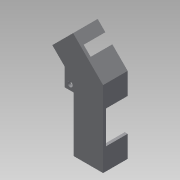
# Autodesk Inventor part: covfronti2c1
Saved by Autodesk Inventor 2015 SP1 (Build 190203100, 203)
## iProperties
Created: 2015-04-15
Part Number: covfronti2c1
Material: Generic
Document SubType Name: Modeling
Designer: Rafi Kurnia Putra
Density: 1 g/cm^3
Appearance: Default
Author: Rafi Kurnia Putra
Autodesk Inventor part; units mm, degrees
ref_plane "YZ Plane" through (0, 0, 0) normal (1, 0, 0) x (0, 1, 0)
ref_plane "XZ Plane" through (0, 0, 0) normal (0, 1, 0) x (-1, 0, 0)
ref_plane "XY Plane" through (0, 0, 0) normal (0, 0, 1) x (1, 0, 0)
sketch "Sketch1" plane through (0, 0, 0) normal (0, 1, 0) x (-1, 0, 0)
  line L0 (-39.6659, 82.3437) -> (-60.406, 61.6036)
  line L1 (-60.406, 61.6036) -> (-60.406, 8.9397)
  circle A0 centre (-37.593, 50.6893) radius 1.75
  circle A1 centre (-37.593, 50.6893) radius 1.75
  line L2 (-60.406, 8.9397) -> (-40.093, 8.9397)
  line L3 (-40.093, 47) -> (-33.9037, 47)
  line L4 (-33.9037, 47) -> (-33.9037, 59.379)
  line L5 (-25.3025, 67.9802) -> (-33.9037, 59.379)
  line L6 (-40.093, 47) -> (-40.093, 8.9397)
  line L7 (-39.6659, 82.3437) -> (-25.3025, 67.9802)
  constraints: 16 end point, 2 centre point, 1 perpendicular
extrude "Extrusion1" add sketch "Sketch1" along normal blind 2
sketch "Sketch2" plane through (0, 2, 0) normal (0, 1, 0) x (1, 0, 0)
  line L0 (39.6659, -82.3437) -> (60.406, -61.6036) projected
  line L1 (60.406, -61.6036) -> (60.406, -8.9397) projected
  line L2 (60.406, -61.6036) -> (60.406, -46.6036)
  line L3 (60.406, -46.6036) -> (58.406, -46.6036)
  line L4 (58.406, -46.6036) -> (58.406, -60.7752)
  line L5 (60.406, -61.6036) -> (49.7994, -72.2102)
  line L6 (49.7994, -72.2102) -> (48.3852, -70.796)
  line L7 (48.3852, -70.796) -> (58.406, -60.7752)
  line L8 (60.406, -8.9397) -> (58.406, -8.9397)
  line L9 (58.406, -8.9397) -> (58.406, -23.9397)
  line L10 (58.406, -23.9397) -> (60.406, -23.9397)
  line L11 (60.406, -23.9397) -> (60.406, -8.9397)
  line L12 (39.6659, -82.3437) -> (44.9692, -77.0404)
  line L13 (44.9692, -77.0404) -> (43.555, -75.6262)
  line L14 (43.555, -75.6262) -> (38.2517, -80.9295)
  line L15 (38.2517, -80.9295) -> (39.6659, -82.3437)
  line L16 (39.6659, -82.3437) -> (47.1659, -82.3437) construction
  point P0 (0, 0)
  dimension "d6" = 15
  dimension "d7" = 2
  dimension "d8" = 15
  dimension "d9" = 2
  dimension "d10" = 90
  dimension "d11" = 90
  dimension "d12" = 15
  dimension "d13" = 7.5
  dimension "d14" = 45
  dimension "d15" = 2
  constraints: 30 end point, 5 perpendicular, 4 parallel, 2 horizontal, 2 point on line, 1 collinear, 1 equal length
  measures "d6" distance of L0.end L2.end
  measures "d7" distance of L2.end L3.end
  measures "d8" distance of L0.end L5.end
  measures "d9" distance of L5.end L6.end
  measures "d10" angle of L5 L6
  measures "d11" angle of L6 L7
  measures "d12" distance of L9.end L8.end
  measures "d13" distance of L0.start L12.end
  measures "d14" angle of L16 L12
  measures "d15" distance of L13.end L12.end
extrude "Extrusion2" add sketch "Sketch2" along normal blind 15
body "Solid1"
